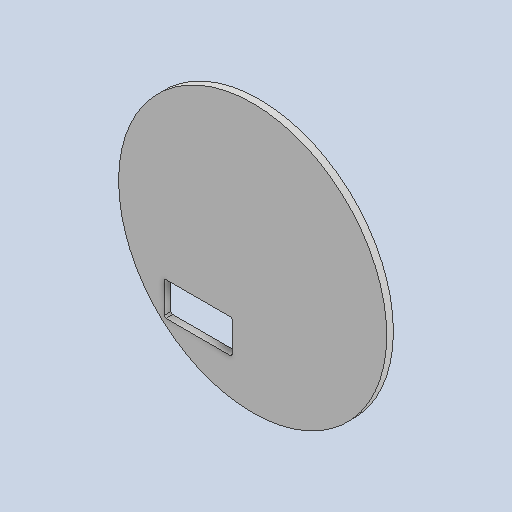
# Autodesk Inventor part: нижний эллипс головы
Saved by Autodesk Inventor 2023.1 (Build 271208000, 208)
## iProperties
Created: 2024-11-21
Part Number: нижний эллипс головы
Material: Типовые
Document SubType Name: Modeling
Designer: DELL
Density: 1 g/cm^3
Appearance: По умолчанию
Author: DELL
Autodesk Inventor part; units mm, degrees
ref_plane "YZ Plane" through (0, 0, 0) normal (1, 0, 0) x (0, 1, 0)
ref_plane "XZ Plane" through (0, 0, 0) normal (0, 1, 0) x (-1, 0, 0)
ref_plane "XY Plane" through (0, 0, 0) normal (0, 0, 1) x (1, 0, 0)
sketch "Эскиз1" plane through (0, 0, 0) normal (0, 0, 1) x (1, 0, 0)
  circle A0 centre (0, 0) radius 80
  line L0 (-52.7593, -38.063) -> (-52.778, -56.063) projected
  line L1 (-14.2583, -37.1029) -> (-50.7583, -37.0651) projected
  line L2 (-12.278, -56.105) -> (-12.2594, -38.105) projected
  line L3 (-50.779, -57.0651) -> (-14.279, -57.1029) projected
  line L4 (-51.7583, -37.063) -> (-13.279, -37.063)
  line L5 (-12.279, -38.063) -> (-12.279, -56.105)
  line L6 (-13.279, -57.105) -> (-51.7583, -57.105)
  line L7 (-52.7583, -56.105) -> (-52.7583, -38.063)
  arc A1 (-52.7583, -56.105) -> (-51.7583, -57.105) centre (-51.7583, -56.105) ccw
  arc A2 (-51.7583, -37.063) -> (-52.7583, -38.063) centre (-51.7583, -38.063) ccw
  arc A3 (-13.279, -57.105) -> (-12.279, -56.105) centre (-13.279, -56.105) ccw
  arc A4 (-12.279, -38.063) -> (-13.279, -37.063) centre (-13.279, -38.063) ccw
  point P0 (-52.7583, -37.063)
  dimension "d2" = 160
  dimension "d3" = 1
  constraints: 8 end point, 8 point on circle, 8 tangent, 5 centre point, 3 equal radius, 3 point on line, 2 parallel, 1 horizontal, 1 perpendicular
  measures "d2" diameter of A0
  measures "d3" radius of A1
extrude "Выдавливание1" add sketch "Эскиз1" against normal blind 4
